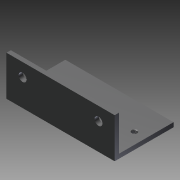
# Autodesk Inventor part: ME5-5
Saved by Autodesk Inventor 2011 SP1 (Build 150282100, 282)
## iProperties
Created: 2015-02-01
Part Number: ME5-5
Catalog Web Link: www.cadenas.de
Description: ME-Magnet Catches for Frames - Plate
Vendor: MISUMI
Document SubType Name: Modeling
Designer: PARTuser1
Manufacturer: MISUMI
Mass: 6.42888 g
Surface Area: 61.7392 cm^2
Volume: 6.42888 cm^3
Density: 1 g/cm^3
Category: PARTsolutions
Company: MISUMI
Title: ME5-5
Author: Cadenas PARTsolutions
Comments: Magnet Catches for Frames - Plate
PSOL_IDENT_0: {\\10.0.0.236\data_v8\23d-libs\misumi\metric\39_accessories_for_al_extrusions\hmgce_plate.prj},148 {
PSOL_IDENT_1: VTYP=3D},{NB=ME5-5},{LINA=ME5-5},{NN=ME},{DATE=17.11.2014 05:31:14},{GEOMDATE=27.07.2009 12:14:00},{
PSOL_IDENT_2: VERSION=},{LINEID=10},{LINESUBID=-1},{WBVAR=}  {NB=ME5-5},{LINA=ME5-5},{KT=DUMMY},{PN=ME5-5},{TYPE=M
PSOL_IDENT_3: E},{NO=5-5},{X=14}
SUPPLIER: MISUMI
ARTICLENO: ME5-5
BOMINFO: ME5-5
CREATOR: CADENAS GmbH
Autodesk Inventor part; units mm, degrees
sketch "Sketch_1" plane through (0, 0, 0) normal (0, 0, 1) x (1, 0, 0)
  line L0 (-28.5, 0) -> (28.5, 0)
  line L1 (28.5, 0) -> (28.5, 31)
  line L2 (28.5, 31) -> (-28.5, 31)
  line L3 (-28.5, 31) -> (-28.5, 0)
  constraints: 8 end point
extrude "Extrusion1" add sketch "Sketch_1" along normal blind 2.3
sketch "Sketch_3" plane through (0, 16.5, 0) normal (0, 1, 0) x (1, 0, 0)
  line L0 (22.5, -2.3) -> (22.5, 0)
  line L1 (22.5, 0) -> (24, 0)
  line L2 (24, 0) -> (23.7295, -0.2705)
  line L3 (23.7295, -0.2705) -> (23.7295, -2.0295)
  line L4 (23.7295, -2.0295) -> (24, -2.3)
  line L5 (24, -2.3) -> (22.5, -2.3)
  line L6 (22.5, -2.3) -> (22.5, 0)
  constraints: 14 end point
revolve "Revolution1" cut sketch "Sketch_3" angle 360 about axis through (22.5, 16.5, 2.3) along (0, 0, 1)
thread "Thread1" size "M3x0.5" class "6H" standard "ISO Metric profile" full length
sketch "Sketch_2" plane through (0, 16.5, 0) normal (0, 1, 0) x (1, 0, 0)
  line L0 (-22.5, -2.3) -> (-22.5, 0)
  line L1 (-22.5, 0) -> (-21, 0)
  line L2 (-21, 0) -> (-21.2705, -0.2705)
  line L3 (-21.2705, -0.2705) -> (-21.2705, -2.0295)
  line L4 (-21.2705, -2.0295) -> (-21, -2.3)
  line L5 (-21, -2.3) -> (-22.5, -2.3)
  line L6 (-22.5, -2.3) -> (-22.5, 0)
  constraints: 14 end point
revolve "Revolution2" cut sketch "Sketch_2" angle 360 about axis through (-22.5, 16.5, 2.3) along (0, 0, 1)
thread "Thread2" size "M3x0.5" class "6H" standard "ISO Metric profile" full length
sketch "Sketch_10" plane through (0, 0, 0) normal (0, 0, 1) x (1, 0, 0)
  line L0 (-28.5, 0) -> (28.5, 0)
  line L1 (28.5, 0) -> (28.5, 2.3)
  line L2 (28.5, 2.3) -> (-28.5, 2.3)
  line L3 (-28.5, 2.3) -> (-28.5, 0)
  constraints: 8 end point
extrude "Extrusion2" add sketch "Sketch_10" along normal blind 21
sketch "Sketch_11" plane through (0, 0, 14) normal (0, 0, 1) x (1, 0, 0)
  line L0 (20, 0) -> (20, 2.3)
  line L1 (20, 2.3) -> (22.1, 2.3)
  line L2 (22.1, 2.3) -> (22.1, 0)
  line L3 (22.1, 0) -> (20, 0)
  line L4 (20, 0) -> (20, 2.3)
  constraints: 10 end point
revolve "Revolution3" cut sketch "Sketch_11" angle 360 about axis through (20, 0, 14) along (0, -1, 0)
sketch "Sketch_12" plane through (0, 0, 14) normal (0, 0, 1) x (1, 0, 0)
  line L0 (-20, 0) -> (-20, 2.3)
  line L1 (-20, 2.3) -> (-17.9, 2.3)
  line L2 (-17.9, 2.3) -> (-17.9, 0)
  line L3 (-17.9, 0) -> (-20, 0)
  line L4 (-20, 0) -> (-20, 2.3)
  constraints: 10 end point
revolve "Revolution4" cut sketch "Sketch_12" angle 360 about axis through (-20, 0, 14) along (0, -1, 0)
ref_plane "mgn_screw1_XY" through (22.5, 16.5, 0) normal (0, 0, 1) x (1, 0, 0)
ref_plane "mgn_screw1_YZ" through (22.5, 16.5, 0) normal (1, 0, 0) x (0, 1, 0)
ref_plane "mgn_screw1_ZX" through (22.5, 16.5, 0) normal (0, 1, 0) x (0, 0, 1)
ref_plane "mgn_screw2_XY" through (-22.5, 16.5, 0) normal (0, 0, 1) x (1, 0, 0)
ref_plane "mgn_screw2_YZ" through (-22.5, 16.5, 0) normal (1, 0, 0) x (0, 1, 0)
ref_plane "mgn_screw2_ZX" through (-22.5, 16.5, 0) normal (0, 1, 0) x (0, 0, 1)
ref_plane "plate_screw1_XY" through (-20, 0, 14) normal (0, 1, 0) x (1, 0, 0)
ref_plane "plate_screw1_YZ" through (-20, 0, 14) normal (1, 0, 0) x (0, 0, -1)
ref_plane "plate_screw1_ZX" through (-20, 0, 14) normal (0, 0, -1) x (0, 1, 0)
ref_plane "plate_screw2_XY" through (20, 0, 14) normal (0, 1, 0) x (1, 0, 0)
ref_plane "plate_screw2_YZ" through (20, 0, 14) normal (1, 0, 0) x (0, 0, -1)
ref_plane "plate_screw2_ZX" through (20, 0, 14) normal (0, 0, -1) x (0, 1, 0)
body "Solid1"
